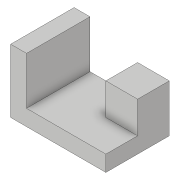
# Autodesk Inventor part: placed_features2
Saved by Autodesk Inventor 2022 Beta2 (Build 260130000, 130) ContinuousBuild 0
## iProperties
Created: 2017-02-06
Part Number: placed_features2
Material: Generic
Document SubType Name: Modeling
Designer: jmacmillan
Density: 1 g/cm^3
Appearance: Default
Author: jmacmillan
Autodesk Inventor part; units mm, degrees
ref_plane "YZ Plane" through (0, 0, 0) normal (1, 0, 0) x (0, 1, 0)
ref_plane "XZ Plane" through (0, 0, 0) normal (0, 1, 0) x (-1, 0, 0)
ref_plane "XY Plane" through (0, 0, 0) normal (0, 0, 1) x (1, 0, 0)
sketch "Sketch1" plane through (0, 0, 0) normal (0, 0, 1) x (1, 0, 0)
  line L0 (0, 101.6) -> (0, 0)
  line L1 (0, 0) -> (152.4, 0)
  line L2 (152.4, 0) -> (152.4, 25.4)
  line L3 (152.4, 25.4) -> (25.4, 25.4)
  line L4 (25.4, 25.4) -> (25.4, 101.6)
  line L5 (25.4, 101.6) -> (0, 101.6)
  dimension "d0" = 76.2
  dimension "d1" = 152.4
  dimension "d2" = 25.4
  constraints: 12 end point, 6 perpendicular, 1 vertical
  measures "d0" distance of L3.end L4.end
  measures "d1" distance of L0.end L1.end
  measures "d2" distance of L1.end L2.end
extrude "Extrusion1" add sketch "Sketch1" against normal blind 101.6
sketch "Sketch2" plane through (25.4, 25.4, 0) normal (0, 1, 0) x (1, 0, 0)
  line L0 (0, 101.6) -> (127, 101.6) projected
  line L1 (127, 0) -> (127, 101.6) projected
  line L2 (76.2, 101.6) -> (76.2, 50.8)
  line L3 (76.2, 50.8) -> (127, 50.8)
  point P0 (-25.4, 0)
  dimension "d5" = 50.8
  dimension "d6" = 50.8
  constraints: 4 end point, 1 midpoint, 1 perpendicular, 1 point on line, 1 vertical
  measures "d5" distance of L2.start L2.end
  measures "d6" distance of L2.end L3.end
extrude "Extrusion2" add sketch "Sketch2" along normal blind 50.8
body "Solid1"
